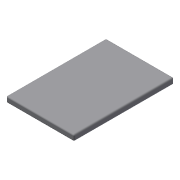
# Autodesk Inventor part: lowerDoor
Saved by Autodesk Inventor 2014 (Build 180170000, 170)
## iProperties
Created: 2014-05-05
Part Number: lowerDoor
Material: 一般
Document SubType Name: Modeling
Designer: motegi
Density: 1 g/cm^3
Appearance: 既定
Author: motegi
Autodesk Inventor part; units mm, degrees
ref_plane "YZ Plane" through (0, 0, 0) normal (1, 0, 0) x (0, 1, 0)
ref_plane "XZ Plane" through (0, 0, 0) normal (0, 1, 0) x (-1, 0, 0)
ref_plane "XY Plane" through (0, 0, 0) normal (0, 0, 1) x (1, 0, 0)
sketch "スケッチ1" plane through (0, 0, 0) normal (0, 0, 1) x (1, 0, 0)
  line L0 (-241, 354.5) -> (241, 354.5)
  line L1 (241, 354.5) -> (241, -354.5)
  line L2 (241, -354.5) -> (-241, -354.5)
  line L3 (-241, -354.5) -> (-241, 354.5)
  line L4 (-241, 354.5) -> (241, -354.5) construction
  line L5 (241, 354.5) -> (-241, -354.5) construction
  point P0 (0, 0)
  dimension "d0" = 482
  dimension "d1" = 709
  constraints: 12 end point, 2 midpoint, 2 parallel, 1 horizontal, 1 perpendicular
  measures "d0" distance of L1.end L2.end
  measures "d1" distance of L0.end L1.end
extrude "押し出し1" add sketch "スケッチ1" along normal blind 43
fillet "フィレット1" radius 10 11 edges at (0, 354.5, 43) (241, 354.5, 21.5) (-241, 354.5, 21.5) (-241, 0, 43) (241, 0, 43) (0, -354.5, 43) (241, -354.5, 21.5) (-241, -354.5, 21.5) (-241, 0, 0) (241, 0, 0) (0, -354.5, 0)
